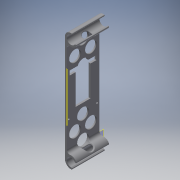
# Autodesk Inventor part: Mount
Saved by Autodesk Inventor 2017 (Build 210142000, 142)
## iProperties
Created: 2017-02-12
Part Number: Mount
Material: Generic
Document SubType Name: Modeling
Designer: Roksbot
Density: 1 g/cm^3
Appearance: Default
Author: Roksbot
Autodesk Inventor part; units mm, degrees
ref_plane "YZ Plane" through (0, 0, 0) normal (1, 0, 0) x (0, 1, 0)
ref_plane "XZ Plane" through (0, 0, 0) normal (0, 1, 0) x (-1, 0, 0)
ref_plane "XY Plane" through (0, 0, 0) normal (0, 0, 1) x (1, 0, 0)
ref_plane "Work Plane1" through (0, 0, 0) normal (0, 0, 1) x (1, 0, 0)
ref_plane "Work Plane2" through (0, -77.4954, -56.8198) normal (0, 0, -1) x (0, 1, 0)
sketch "Sketch1" plane through (0, 0, 0) normal (0, 0, 1) x (1, 0, 0)
  line L0 (6.0738, -139.5414) -> (7.874, -140.5807) construction
  line L1 (7.874, -140.5807) -> (9.6742, -139.5414) construction
  arc A0 (12.4238, -137.9539) -> (9.6742, -139.5414) centre (11.049, -138.7477) ccw construction
  line L2 (12.4238, -137.9539) -> (14.224, -136.9146) construction
  line L3 (14.224, -136.9146) -> (14.224, -134.8359) construction
  arc A1 (14.224, -131.6609) -> (14.224, -134.8359) centre (14.224, -133.2484) ccw construction
  line L4 (14.224, -131.6609) -> (14.224, -129.5822) construction
  line L5 (14.224, -129.5822) -> (12.4238, -128.5429) construction
  arc A2 (9.6742, -126.9554) -> (12.4238, -128.5429) centre (11.049, -127.7491) ccw construction
  line L6 (9.6742, -126.9554) -> (7.874, -125.9161) construction
  line L7 (7.874, -125.9161) -> (6.0738, -126.9554) construction
  arc A3 (3.3242, -128.5429) -> (6.0738, -126.9554) centre (4.699, -127.7491) ccw construction
  line L8 (3.3242, -128.5429) -> (1.524, -129.5822) construction
  line L9 (1.524, -129.5822) -> (1.524, -131.6609) construction
  arc A4 (1.524, -134.8359) -> (1.524, -131.6609) centre (1.524, -133.2484) ccw construction
  line L10 (1.524, -134.8359) -> (1.524, -136.9146) construction
  line L11 (1.524, -136.9146) -> (3.3242, -137.9539) construction
  arc A5 (6.0738, -139.5414) -> (3.3242, -137.9539) centre (4.699, -138.7477) ccw construction
  circle A6 centre (7.874, -133.2484) radius 2.9337 construction
  line L12 (6.0738, 44.6086) -> (7.874, 43.5693) construction
  line L13 (7.874, 43.5693) -> (9.6742, 44.6086) construction
  arc A7 (12.4238, 46.1961) -> (9.6742, 44.6086) centre (11.049, 45.4023) ccw construction
  line L14 (12.4238, 46.1961) -> (14.224, 47.2354) construction
  line L15 (14.224, 47.2354) -> (14.224, 49.3141) construction
  arc A8 (14.224, 52.4891) -> (14.224, 49.3141) centre (14.224, 50.9016) ccw construction
  line L16 (14.224, 52.4891) -> (14.224, 54.5678) construction
  line L17 (14.224, 54.5678) -> (12.4238, 55.6071) construction
  arc A9 (9.6742, 57.1946) -> (12.4238, 55.6071) centre (11.049, 56.4009) ccw construction
  line L18 (9.6742, 57.1946) -> (7.874, 58.2339) construction
  line L19 (7.874, 58.2339) -> (6.0738, 57.1946) construction
  arc A10 (3.3242, 55.6071) -> (6.0738, 57.1946) centre (4.699, 56.4009) ccw construction
  line L20 (3.3242, 55.6071) -> (1.524, 54.5678) construction
  line L21 (1.524, 54.5678) -> (1.524, 52.4891) construction
  arc A11 (1.524, 49.3141) -> (1.524, 52.4891) centre (1.524, 50.9016) ccw construction
  line L22 (1.524, 49.3141) -> (1.524, 47.2354) construction
  line L23 (1.524, 47.2354) -> (3.3242, 46.1961) construction
  arc A12 (6.0738, 44.6086) -> (3.3242, 46.1961) centre (4.699, 45.4023) ccw construction
  circle A13 centre (7.874, 50.9016) radius 2.9337 construction
  line L24 (0, -77.4954) -> (0, 0) construction
  line L25 (0, -77.4954) -> (1.524, -77.4954) construction
  line L26 (1.524, 0) -> (1.524, -77.4954) construction
  line L27 (0, 0) -> (1.524, 0) construction
  line L28 (1.6256, -60.0964) -> (8.7376, -60.0964) construction
  line L29 (8.7376, -22.2504) -> (1.6256, -22.2504) construction
  line L30 (0, -7.62) -> (-9.779, -7.62) construction
  line L31 (0, -2.54) -> (-9.779, -2.54) construction
  arc A14 (14.2678, -129.6075) -> (7.9178, -140.606) centre (7.874, -133.2484) ccw
  arc A15 (7.9178, 58.2592) -> (14.2678, 47.2607) centre (7.874, 50.9016) ccw
  arc A16 (11.9765, 60.6025) -> (18.3265, 49.604) centre (7.874, 50.9016) ccw
  arc A17 (18.3265, -131.9508) -> (11.9765, -142.9493) centre (7.874, -133.2484) ccw
  circle A18 centre (7.874, -133.2484) radius 7.3323 construction
  line L32 (14.8793, -41.1734) -> (-13.8887, -41.1734) construction
  line L33 (11.9765, -142.9493) -> (7.9178, -140.606)
  line L34 (18.3265, -131.9508) -> (14.2678, -129.6075)
  line L35 (14.2678, 47.2607) -> (18.3265, 49.604)
  line L36 (7.9178, 58.2592) -> (11.9765, 60.6025)
  line L37 (0.5163, -133.2484) -> (0.5163, 50.9016)
  line L38 (-2.6587, -133.2484) -> (-2.6587, 50.9016)
extrude "Extrusion1" add sketch "Sketch1" against normal up to surface (56.8198 mm away)
fillet "Fillet1" radius 1.27 8 edges at (18.3265, -131.9508, -28.4099) (14.2678, -129.6075, -28.4099) (11.9765, -142.9493, -28.4099) (7.9178, -140.606, -28.4099) (18.3265, 49.604, -28.4099) (14.2678, 47.2607, -28.4099) (11.9765, 60.6025, -28.4099) (7.9178, 58.2592, -28.4099)
fillet "Fillet2" radius 5.08 2 edges at (0.5163, 43.3649, -28.4099) (0.5163, -125.7117, -28.4099)
ref_plane "Work Plane3" through (-2.3793, -133.2484, -56.1848) normal (-1, 0, 0) x (0, 0, 1)
sketch "Sketch2" plane through (-2.3793, -133.2484, -56.1848) normal (-1, 0, 0) x (0, 0, 1)
  circle A0 centre (3.1496, 59.436) radius 1.5875 projected
  circle A1 centre (52.4002, 59.436) radius 1.5875 projected
  point P0 (56.1848, 133.2484)
extrude "Extrusion2" cut sketch "Sketch2" against normal through all
sketch "Sketch3" plane through (-2.6587, -133.2484, 0) normal (-1, 0, 0) x (0, 0, 1)
  line L0 (-34.544, 73.152) -> (-22.2758, 73.152) construction
  line L1 (-40.259, 101.854) -> (-40.259, 79.502) construction
  line L2 (-16.5608, 79.502) -> (-16.5608, 101.854) construction
  line L3 (-50.3174, 125.6284) -> (-6.5024, 125.6284) construction
  line L4 (-6.5024, 125.6284) -> (-6.5024, 130.7084) construction
  line L5 (-6.5024, 130.7084) -> (-50.3174, 130.7084) construction
  line L6 (-50.3174, 130.7084) -> (-50.3174, 125.6284) construction
  line L7 (-41.529, 124.3584) -> (-15.2908, 124.3584)
  line L8 (-15.2908, 124.3584) -> (-15.2908, 71.882)
  line L9 (-15.2908, 71.882) -> (-41.529, 71.882)
  line L10 (-41.529, 71.882) -> (-41.529, 124.3584)
  line L11 (-41.529, 124.3584) -> (-15.2908, 71.882) construction
  line L12 (-15.2908, 124.3584) -> (-41.529, 71.882) construction
  line L13 (-51.5874, 131.9784) -> (-5.2324, 131.9784)
  line L14 (-5.2324, 131.9784) -> (-5.2324, 124.3584)
  line L15 (-5.2324, 124.3584) -> (-51.5874, 124.3584)
  line L16 (-51.5874, 124.3584) -> (-51.5874, 131.9784)
  line L17 (-51.5874, 131.9784) -> (-5.2324, 124.3584) construction
  line L18 (-5.2324, 131.9784) -> (-51.5874, 124.3584) construction
  point P0 (0, 133.2484)
  point P1 (-28.4099, 98.1202)
  point P2 (-28.4099, 128.1684)
  point P3 (-28.4099, 128.1684)
  point P4 (-28.4099, 125.6284)
  point P5 (-28.4099, 98.1202)
  point P6 (-28.4099, 98.1202)
  point P7 (-28.4099, 73.152)
  dimension "d9" = 1.27
  dimension "d10" = 1.27
  dimension "d11" = 1.27
  dimension "d12" = 1.27
  dimension "d13" = 1.27
  constraints: 24 end point, 9 midpoint, 4 parallel, 2 horizontal, 2 perpendicular, 2 vertical alignment, 1 coincident, 1 point on line
  measures "d9" distance between parallel lines of L1 L10
  measures "d10" distance between parallel lines of L0 L9
  measures "d11" distance between parallel lines of L6 L16
  measures "d12" distance between parallel lines of L5 L13
  measures "d13" distance between parallel lines of L3 L7
extrude "Extrusion3" cut sketch "Sketch3" against normal through all
sketch "Sketch4" plane through (-2.6587, -133.2484, 0) normal (-1, 0, 0) x (0, 0, 1)
  circle A0 centre (-28.4099, 15.4457) radius 9.525
  circle A1 centre (-42.2148, 35.2367) radius 9.525
  circle A2 centre (-28.4099, 55.0276) radius 9.525
  circle A3 centre (-14.605, 35.2367) radius 9.525
  circle A4 centre (-28.4099, 129.1224) radius 9.525
  circle A5 centre (-42.2148, 148.9133) radius 9.525
  circle A6 centre (-28.4099, 168.7043) radius 9.525
  circle A7 centre (-14.605, 148.9133) radius 9.525
  line L0 (39.7002, 92.075) -> (-124.7648, 92.075) construction
  line L1 (-28.4099, 15.4457) -> (-42.2148, 35.2367) construction
  line L2 (-42.2148, 35.2367) -> (-28.4099, 55.0276) construction
  line L3 (-28.4099, 55.0276) -> (-14.605, 35.2367) construction
  line L4 (-14.605, 35.2367) -> (-28.4099, 15.4457) construction
  line L5 (0, -10.5327) -> (-56.8198, -10.5327) construction
  line L6 (-56.8198, 184.15) -> (-56.8198, 0) construction
  line L7 (-56.8198, 15.4457) -> (0, 15.4457) construction
  point P0 (0, 133.2484)
  point P1 (-28.4099, -10.5327)
  dimension "d16" = 19.05
  dimension "d17" = 5.08
  dimension "d18" = 5.08
  constraints: 10 end point, 8 centre point, 7 equal radius, 6 vertical alignment, 2 horizontal alignment, 2 midpoint, 1 equal length, 1 horizontal, 1 parallel, 6 other
  measures "d16" diameter of A1
  measures "d18" distance edge to line of A1 L6
extrude "Extrusion4" cut sketch "Sketch4" against normal through all
fillet "Fillet4" radius 1.27 20 edges at (0.5163, -98.0117, -51.7398) (-2.6587, -98.0117, -51.7398) (-2.6587, -78.2208, -37.9349) (0.5163, -78.2208, -37.9349) (-2.6587, -98.0117, -24.13) (0.5163, -98.0117, -24.13) (-2.6587, -117.8027, -37.9349) (2.595, -121.9013, -37.008) (16.5851, -127.3277, -28.4103) (2.595, -121.9013, -19.8118) (0.5163, -108.2777, -28.4099) (-2.6587, 15.6649, -51.7398) (0.5163, 15.6649, -51.7398) (-2.6587, 35.4559, -37.9349) (2.595, 39.5545, -19.8118) (16.5851, 44.9809, -28.4095) (2.595, 39.5545, -37.008) (0.5163, 25.9309, -28.4099) (-2.6587, 15.6649, -24.13) (0.5163, 15.6649, -24.13)
fillet "Fillet5" radius 1.27 2 edges at (3.5057, -127.3277, -28.4099) (12.2423, 44.9809, -28.4099)
sketch "Sketch5" plane through (0, 0, 0) normal (0, 0, 1) x (1, 0, 0)
  line L0 (-16.5783, -152.6745) -> (22.1686, -152.6745)
  line L1 (22.1686, -152.6745) -> (22.1686, -117.5902)
  line L2 (22.1686, -117.5902) -> (-16.5783, -117.5902)
  line L3 (-16.5783, -117.5902) -> (-16.5783, -152.6745)
  point P0 (0, 0)
  constraints: 8 end point, 2 parallel, 1 horizontal, 1 perpendicular
extrude "Extrusion5" [suppressed]
equation "\"d13\" = d12"
equation "\"d18\" = d17"
body "Solid1"
